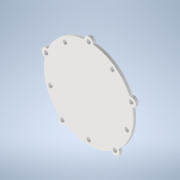
# Autodesk Inventor part: Base_Suelo
Saved by Autodesk Inventor 2022 (Build 260153000, 153)
## iProperties
Created: 2021-09-09
Part Number: Base_Suelo
Material: Generic
Document SubType Name: Modeling
Designer: Administrador
Density: 1 g/cm^3
Appearance: Default
Author: Administrador
Autodesk Inventor part; units mm, degrees
ref_plane "YZ Plane" through (0, 0, 0) normal (1, 0, 0) x (0, 1, 0)
ref_plane "XZ Plane" through (0, 0, 0) normal (0, 1, 0) x (-1, 0, 0)
ref_plane "XY Plane" through (0, 0, 0) normal (0, 0, 1) x (1, 0, 0)
sketch "Sketch1" plane through (0, 0, 0) normal (0, 1, 0) x (-1, 0, 0)
  point P0 (0, 0)
sketch "Sketch2" plane through (0, 0, 0) normal (0, 0, 1) x (1, 0, 0)
  line L0 (0, -49) -> (0, -44)
  circle A0 centre (0, -44) radius 2.4
  circle A1 centre (-41.8465, -13.5967) radius 2.4
  circle A2 centre (-25.8626, 35.5967) radius 2.4
  circle A3 centre (25.8626, 35.5967) radius 2.4
  circle A4 centre (41.8465, -13.5967) radius 2.4
  arc A5 (4.9935, 48.7449) -> (-4.9935, 48.7449) centre (0, 49) ccw
  circle A6 centre (0, 49) radius 2.4
  arc A7 (0, 49) -> (-2.3993, 48.9412) centre (0, 0) ccw
  arc A8 (-2.3991, -43.9345) -> (0, -44) centre (0, 0) ccw
  arc A9 (-44.8161, 19.8121) -> (-47.9022, 10.3139) centre (-46.6018, 15.1418) ccw
  circle A10 centre (-46.6018, 15.1418) radius 2.4
  arc A11 (-32.6913, -36.5004) -> (-24.6117, -42.3705) centre (-28.8015, -39.6418) ccw
  circle A12 centre (-28.8015, -39.6418) radius 2.4
  arc A13 (24.6117, -42.3705) -> (32.6913, -36.5004) centre (28.8015, -39.6418) ccw
  circle A14 centre (28.8015, -39.6418) radius 2.4
  arc A15 (47.9022, 10.3139) -> (44.8161, 19.8121) centre (46.6018, 15.1418) ccw
  circle A16 centre (46.6018, 15.1418) radius 2.4
  arc A17 (-4.9935, 48.7449) -> (-44.8161, 19.8121) centre (0, 0) ccw
  arc A18 (-47.9022, 10.3139) -> (-32.6913, -36.5004) centre (0, 0) ccw
  arc A19 (-24.6117, -42.3705) -> (24.6117, -42.3705) centre (0, 0) ccw
  arc A20 (32.6913, -36.5004) -> (47.9022, 10.3139) centre (0, 0) ccw
  arc A21 (44.8161, 19.8121) -> (4.9935, 48.7449) centre (0, 0) ccw
  point P0 (2.3993, 48.9412)
  point P1 (-47.2873, 12.8418)
  point P2 (-45.8045, 17.4055)
  point P3 (-30.708, -38.184)
  point P4 (26.8259, -41.0045)
  point P5 (47.2873, 12.8418)
  point P6 (-26.8259, -41.0045)
  point P7 (30.708, -38.184)
  point P8 (45.8045, 17.4055)
  dimension "d2" = 4.8
  dimension "d1" = 5
  dimension "d5" = 360
  dimension "d7" = 10
  dimension "d8" = 4.8
  dimension "d11" = 360
  constraints: 35 point on circle, 21 centre point, 8 coincident, 2 end point, 1 point on line, 1 vertical, 55 other
  measures "d1" distance of L0.end L0.start
  measures "d7" diameter of A5
  measures "d8" diameter of A6
extrude "BaseSuelo" add sketch "Sketch2" along normal blind 3
body "Solid1"
